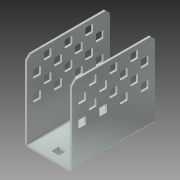
# Autodesk Inventor part: 276-1926
Saved by Autodesk Inventor 2013 (Build 170138000, 138)
## iProperties
Category: Motion
Company: Autodesk Inc.
Created: 2012-02-28
Part Number: 276-1926
Material: Steel
Document SubType Name: Sheet Metal
Designer: Autodesk Inc.
Density: 7.85 g/cm^3
Sheet Metal Rule: Default
Catalog Web Link: http://www.vexrobotics.com/276-1926.html
Vendor: VEX
Author: Autodesk Inc.
Autodesk Inventor part; units mm, degrees
ref_plane "YZ Plane" through (0, 0, 0) normal (1, 0, 0) x (0, 1, 0)
ref_plane "XZ Plane" through (0, 0, 0) normal (0, 1, 0) x (-1, 0, 0)
ref_plane "XY Plane" through (0, 0, 0) normal (0, 0, 1) x (1, 0, 0)
sketch "Sketch1" plane through (0, 0, 0) normal (0, 0, 1) x (1, 0, 0)
  line L0 (0, 0) -> (50.8, 0)
  line L1 (50.8, 0) -> (50.8, 28.6766)
  line L2 (50.8, 28.6766) -> (0, 28.6766)
  line L3 (0, 28.6766) -> (0, 0)
  dimension "d0" = 50.8
  dimension "d1" = 28.6766
  measures "d0" distance of L2.end L1.end
  measures "d1" distance of L1.end L0.end
extrude "Plate1" add sketch "Sketch1" against normal blind 1.19
sketch "Sketch2" plane through (50.8, 1.19, -1.19) normal (0, -1, 0) x (1, 0, 0)
  line L0 (-50.8, 0) -> (0, 0)
  line L1 (0, 0) -> (0, 47.879)
  line L2 (0, 47.879) -> (-50.8, 47.879)
  line L3 (-50.8, 47.879) -> (-50.8, 0)
  constraints: 6 end point, 1 horizontal, 1 perpendicular, 1 vertical
edge flange "Flange1" height 47.879 angle 90 thickness 1.19 bend radius 1.19 thickness toward (0, -1, 0) relief straight relief width 1.19 relief depth 0.595 corner gap 1.19 corner form 0 edges at (25.4, 0, 0) (25.4, 28.6766, 0) wall of the first edge with corners at (0, 1.19, -1.19) (50.8, 1.19, -1.19) (50.8, 1.19, 46.689) (0, 1.19, 46.689)
bend "Bend1"
corner "Corner1"
chamfer "Corner Chamfer1" distance 2.54 angle 45 4 edges at (0, 28.0816, 46.689) (0, 0.595, 46.689) (50.8, 28.0816, 46.689) (50.8, 0.595, 46.689)
sketch "Sketch3" plane through (0, 0, 1.19) normal (0, -1, 0) x (1, 0, 0)
  line L0 (2.54, 45.499) -> (48.26, 45.499) projected
  line L1 (0, 0) -> (0, 42.959) projected
  line L2 (10.8966, 37.9552) -> (14.5034, 37.9552)
  line L3 (15.0114, 38.4632) -> (15.0114, 42.07)
  line L4 (14.5034, 42.578) -> (10.8966, 42.578)
  line L5 (10.3886, 42.07) -> (10.3886, 38.4632)
  line L6 (12.7, 37.9552) -> (12.7, 42.578) construction
  line L7 (10.3886, 40.2666) -> (15.0114, 40.2666) construction
  arc A0 (10.8966, 42.578) -> (10.3886, 42.07) centre (10.8966, 42.07) ccw
  arc A1 (15.0114, 42.07) -> (14.5034, 42.578) centre (14.5034, 42.07) ccw
  arc A2 (14.5034, 37.9552) -> (15.0114, 38.4632) centre (14.5034, 38.4632) ccw
  arc A3 (10.3886, 38.4632) -> (10.8966, 37.9552) centre (10.8966, 38.4632) ccw
  line L8 (23.5966, 37.9552) -> (27.2034, 37.9552)
  line L9 (27.7114, 38.4632) -> (27.7114, 42.07)
  line L10 (27.2034, 42.578) -> (23.5966, 42.578)
  line L11 (23.0886, 42.07) -> (23.0886, 38.4632)
  line L12 (25.4, 37.9552) -> (25.4, 42.578) construction
  line L13 (23.0886, 40.2666) -> (27.7114, 40.2666) construction
  arc A4 (23.5966, 42.578) -> (23.0886, 42.07) centre (23.5966, 42.07) ccw
  arc A5 (27.7114, 42.07) -> (27.2034, 42.578) centre (27.2034, 42.07) ccw
  arc A6 (27.2034, 37.9552) -> (27.7114, 38.4632) centre (27.2034, 38.4632) ccw
  arc A7 (23.0886, 38.4632) -> (23.5966, 37.9552) centre (23.5966, 38.4632) ccw
  line L14 (36.2966, 37.9552) -> (39.9034, 37.9552)
  line L15 (40.4114, 38.4632) -> (40.4114, 42.07)
  line L16 (39.9034, 42.578) -> (36.2966, 42.578)
  line L17 (35.7886, 42.07) -> (35.7886, 38.4632)
  line L18 (38.1, 37.9552) -> (38.1, 42.578) construction
  line L19 (35.7886, 40.2666) -> (40.4114, 40.2666) construction
  arc A8 (36.2966, 42.578) -> (35.7886, 42.07) centre (36.2966, 42.07) ccw
  arc A9 (40.4114, 42.07) -> (39.9034, 42.578) centre (39.9034, 42.07) ccw
  arc A10 (39.9034, 37.9552) -> (40.4114, 38.4632) centre (39.9034, 38.4632) ccw
  arc A11 (35.7886, 38.4632) -> (36.2966, 37.9552) centre (36.2966, 38.4632) ccw
  line L20 (10.8966, 25.2552) -> (14.5034, 25.2552)
  line L21 (15.0114, 25.7632) -> (15.0114, 29.37)
  line L22 (14.5034, 29.878) -> (10.8966, 29.878)
  line L23 (10.3886, 29.37) -> (10.3886, 25.7632)
  line L24 (12.7, 25.2552) -> (12.7, 29.878) construction
  line L25 (10.3886, 27.5666) -> (15.0114, 27.5666) construction
  arc A12 (10.8966, 29.878) -> (10.3886, 29.37) centre (10.8966, 29.37) ccw
  arc A13 (15.0114, 29.37) -> (14.5034, 29.878) centre (14.5034, 29.37) ccw
  arc A14 (14.5034, 25.2552) -> (15.0114, 25.7632) centre (14.5034, 25.7632) ccw
  arc A15 (10.3886, 25.7632) -> (10.8966, 25.2552) centre (10.8966, 25.7632) ccw
  line L26 (23.5966, 25.2552) -> (27.2034, 25.2552)
  line L27 (27.7114, 25.7632) -> (27.7114, 29.37)
  arc A16 (23.0886, 25.7632) -> (23.5966, 25.2552) centre (23.5966, 25.7632) ccw
  arc A17 (27.7114, 29.37) -> (27.2034, 29.878) centre (27.2034, 29.37) ccw
  line L28 (23.0886, 27.5666) -> (27.7114, 27.5666) construction
  line L29 (25.4, 25.2552) -> (25.4, 29.878) construction
  line L30 (23.0886, 29.37) -> (23.0886, 25.7632)
  arc A18 (23.5966, 29.878) -> (23.0886, 29.37) centre (23.5966, 29.37) ccw
  arc A19 (27.2034, 25.2552) -> (27.7114, 25.7632) centre (27.2034, 25.7632) ccw
  line L31 (27.2034, 29.878) -> (23.5966, 29.878)
  line L32 (36.2966, 25.2552) -> (39.9034, 25.2552)
  line L33 (40.4114, 25.7632) -> (40.4114, 29.37)
  arc A20 (35.7886, 25.7632) -> (36.2966, 25.2552) centre (36.2966, 25.7632) ccw
  arc A21 (40.4114, 29.37) -> (39.9034, 29.878) centre (39.9034, 29.37) ccw
  line L34 (35.7886, 27.5666) -> (40.4114, 27.5666) construction
  line L35 (38.1, 25.2552) -> (38.1, 29.878) construction
  line L36 (35.7886, 29.37) -> (35.7886, 25.7632)
  arc A22 (36.2966, 29.878) -> (35.7886, 29.37) centre (36.2966, 29.37) ccw
  arc A23 (39.9034, 25.2552) -> (40.4114, 25.7632) centre (39.9034, 25.7632) ccw
  line L37 (39.9034, 29.878) -> (36.2966, 29.878)
  line L38 (4.5466, 31.6052) -> (8.1534, 31.6052)
  line L39 (8.6614, 32.1132) -> (8.6614, 35.72)
  line L40 (8.1534, 36.228) -> (4.5466, 36.228)
  line L41 (4.0386, 35.72) -> (4.0386, 32.1132)
  arc A24 (4.0386, 32.1132) -> (4.5466, 31.6052) centre (4.5466, 32.1132) ccw
  arc A25 (4.5466, 36.228) -> (4.0386, 35.72) centre (4.5466, 35.72) ccw
  arc A26 (8.6614, 35.72) -> (8.1534, 36.228) centre (8.1534, 35.72) ccw
  arc A27 (8.1534, 31.6052) -> (8.6614, 32.1132) centre (8.1534, 32.1132) ccw
  line L42 (6.35, 31.6052) -> (6.35, 36.228) construction
  line L43 (4.0386, 33.9166) -> (8.6614, 33.9166) construction
  line L44 (17.2466, 31.6052) -> (20.8534, 31.6052)
  line L45 (21.3614, 32.1132) -> (21.3614, 35.72)
  line L46 (20.8534, 36.228) -> (17.2466, 36.228)
  line L47 (16.7386, 35.72) -> (16.7386, 32.1132)
  arc A28 (16.7386, 32.1132) -> (17.2466, 31.6052) centre (17.2466, 32.1132) ccw
  arc A29 (17.2466, 36.228) -> (16.7386, 35.72) centre (17.2466, 35.72) ccw
  arc A30 (21.3614, 35.72) -> (20.8534, 36.228) centre (20.8534, 35.72) ccw
  arc A31 (20.8534, 31.6052) -> (21.3614, 32.1132) centre (20.8534, 32.1132) ccw
  line L48 (19.05, 31.6052) -> (19.05, 36.228) construction
  line L49 (16.7386, 33.9166) -> (21.3614, 33.9166) construction
  line L50 (29.9466, 31.6052) -> (33.5534, 31.6052)
  line L51 (34.0614, 32.1132) -> (34.0614, 35.72)
  line L52 (33.5534, 36.228) -> (29.9466, 36.228)
  line L53 (29.4386, 35.72) -> (29.4386, 32.1132)
  arc A32 (29.4386, 32.1132) -> (29.9466, 31.6052) centre (29.9466, 32.1132) ccw
  arc A33 (29.9466, 36.228) -> (29.4386, 35.72) centre (29.9466, 35.72) ccw
  arc A34 (34.0614, 35.72) -> (33.5534, 36.228) centre (33.5534, 35.72) ccw
  arc A35 (33.5534, 31.6052) -> (34.0614, 32.1132) centre (33.5534, 32.1132) ccw
  line L54 (31.75, 31.6052) -> (31.75, 36.228) construction
  line L55 (29.4386, 33.9166) -> (34.0614, 33.9166) construction
  line L56 (42.6466, 31.6052) -> (46.2534, 31.6052)
  line L57 (46.7614, 32.1132) -> (46.7614, 35.72)
  line L58 (46.2534, 36.228) -> (42.6466, 36.228)
  line L59 (42.1386, 35.72) -> (42.1386, 32.1132)
  arc A36 (42.1386, 32.1132) -> (42.6466, 31.6052) centre (42.6466, 32.1132) ccw
  arc A37 (42.6466, 36.228) -> (42.1386, 35.72) centre (42.6466, 35.72) ccw
  arc A38 (46.7614, 35.72) -> (46.2534, 36.228) centre (46.2534, 35.72) ccw
  arc A39 (46.2534, 31.6052) -> (46.7614, 32.1132) centre (46.2534, 32.1132) ccw
  line L60 (44.45, 31.6052) -> (44.45, 36.228) construction
  line L61 (42.1386, 33.9166) -> (46.7614, 33.9166) construction
  line L62 (4.5466, 18.9052) -> (8.1534, 18.9052)
  line L63 (8.6614, 19.4132) -> (8.6614, 23.02)
  line L64 (8.1534, 23.528) -> (4.5466, 23.528)
  line L65 (4.0386, 23.02) -> (4.0386, 19.4132)
  arc A40 (4.0386, 19.4132) -> (4.5466, 18.9052) centre (4.5466, 19.4132) ccw
  arc A41 (4.5466, 23.528) -> (4.0386, 23.02) centre (4.5466, 23.02) ccw
  arc A42 (8.6614, 23.02) -> (8.1534, 23.528) centre (8.1534, 23.02) ccw
  arc A43 (8.1534, 18.9052) -> (8.6614, 19.4132) centre (8.1534, 19.4132) ccw
  line L66 (6.35, 18.9052) -> (6.35, 23.528) construction
  line L67 (4.0386, 21.2166) -> (8.6614, 21.2166) construction
  line L68 (17.2466, 18.9052) -> (20.8534, 18.9052)
  line L69 (21.3614, 19.4132) -> (21.3614, 23.02)
  line L70 (20.8534, 23.528) -> (17.2466, 23.528)
  line L71 (16.7386, 23.02) -> (16.7386, 19.4132)
  arc A44 (16.7386, 19.4132) -> (17.2466, 18.9052) centre (17.2466, 19.4132) ccw
  arc A45 (17.2466, 23.528) -> (16.7386, 23.02) centre (17.2466, 23.02) ccw
  arc A46 (21.3614, 23.02) -> (20.8534, 23.528) centre (20.8534, 23.02) ccw
  arc A47 (20.8534, 18.9052) -> (21.3614, 19.4132) centre (20.8534, 19.4132) ccw
  line L72 (19.05, 18.9052) -> (19.05, 23.528) construction
  line L73 (16.7386, 21.2166) -> (21.3614, 21.2166) construction
  line L74 (29.9466, 18.9052) -> (33.5534, 18.9052)
  line L75 (34.0614, 19.4132) -> (34.0614, 23.02)
  line L76 (33.5534, 23.528) -> (29.9466, 23.528)
  line L77 (29.4386, 23.02) -> (29.4386, 19.4132)
  arc A48 (29.4386, 19.4132) -> (29.9466, 18.9052) centre (29.9466, 19.4132) ccw
  arc A49 (29.9466, 23.528) -> (29.4386, 23.02) centre (29.9466, 23.02) ccw
  arc A50 (34.0614, 23.02) -> (33.5534, 23.528) centre (33.5534, 23.02) ccw
  arc A51 (33.5534, 18.9052) -> (34.0614, 19.4132) centre (33.5534, 19.4132) ccw
  line L78 (31.75, 18.9052) -> (31.75, 23.528) construction
  line L79 (29.4386, 21.2166) -> (34.0614, 21.2166) construction
  line L80 (42.6466, 18.9052) -> (46.2534, 18.9052)
  line L81 (46.7614, 19.4132) -> (46.7614, 23.02)
  line L82 (46.2534, 23.528) -> (42.6466, 23.528)
  line L83 (42.1386, 23.02) -> (42.1386, 19.4132)
  arc A52 (42.1386, 19.4132) -> (42.6466, 18.9052) centre (42.6466, 19.4132) ccw
  arc A53 (42.6466, 23.528) -> (42.1386, 23.02) centre (42.6466, 23.02) ccw
  arc A54 (46.7614, 23.02) -> (46.2534, 23.528) centre (46.2534, 23.02) ccw
  arc A55 (46.2534, 18.9052) -> (46.7614, 19.4132) centre (46.2534, 19.4132) ccw
  line L84 (44.45, 18.9052) -> (44.45, 23.528) construction
  line L85 (42.1386, 21.2166) -> (46.7614, 21.2166) construction
  point P0 (0, -1.19)
  point P1 (15.0114, 42.578)
  point P2 (15.0114, 37.9552)
  point P3 (10.3886, 42.578)
  point P4 (27.7114, 42.578)
  point P5 (27.7114, 37.9552)
  point P6 (23.0886, 42.578)
  point P7 (40.4114, 42.578)
  point P8 (40.4114, 37.9552)
  point P9 (35.7886, 42.578)
  point P10 (15.0114, 29.878)
  point P11 (15.0114, 25.2552)
  point P12 (10.3886, 29.878)
  point P13 (27.7114, 25.2552)
  point P14 (27.7114, 29.878)
  point P15 (23.0886, 29.878)
  point P16 (40.4114, 25.2552)
  point P17 (40.4114, 29.878)
  point P18 (35.7886, 29.878)
  dimension "d16" = 4.6228
  dimension "d17" = 4.6228
  dimension "d18" = 0.508
  dimension "d19" = 12.7
  dimension "d20" = 5.2324
  dimension "d23" = 12.7
  dimension "d30" = 12.7
  dimension "d35" = 0.508
  dimension "d36" = 6.35
  dimension "d37" = 4.6228
  dimension "d38" = 4.6228
  dimension "d39" = 6.35
  dimension "d42" = 12.7
  dimension "d45" = 12.7
  constraints: 168 end point, 112 point on circle, 56 centre point, 36 point on line, 16 tangent, 8 midpoint, 6 equal radius, 4 horizontal, 4 parallel, 2 perpendicular, 2 vertical, 327 other
  measures "d16" distance of point (10.389, 42.578) point (15.011, 42.578)
  measures "d17" distance of point (15.011, 42.578) point (15.011, 37.955)
  measures "d18" radius of A0
  measures "d19" distance between parallel lines of L6 L1
  measures "d20" distance between parallel lines of L7 L0
  measures "d23" distance of point (15.011, 37.955) point (27.711, 37.955)
  measures "d30" distance of L4.start L22.start
  measures "d35" radius of A24
  measures "d36" distance between parallel lines of L42 L1
  measures "d37" distance between parallel lines of L38 L40
  measures "d38" distance between parallel lines of L39 L41
  measures "d39" distance between parallel lines of L43 L7
  measures "d42" distance of L39.end L45.end
  measures "d45" distance of L39.end L63.end
extrude "Cut1" cut sketch "Sketch3" against normal blind 1.19
ref_plane "Work Plane1" through (0, 14.3383, 1.19) normal (0, -1, 0) x (1, 0, 0)
mirror "Mirror1" about plane through (0, 14.3383, 1.19) normal (0, -1, 0) of "Cut1"
sketch "Sketch4" plane through (0, 0, -1.19) normal (0, 0, -1) x (-1, 0, 0)
  line L0 (-50.8, 2.38) -> (0, 2.38) projected
  line L1 (0, 26.2966) -> (0, 2.38) projected
  line L2 (-4.5466, 16.6497) -> (-8.1534, 16.6497)
  line L3 (-8.6614, 16.1417) -> (-8.6614, 12.5349)
  line L4 (-8.1534, 12.0269) -> (-4.5466, 12.0269)
  line L5 (-4.0386, 12.5349) -> (-4.0386, 16.1417)
  arc A0 (-4.5466, 12.0269) -> (-4.0386, 12.5349) centre (-4.5466, 12.5349) ccw
  arc A1 (-8.6614, 12.5349) -> (-8.1534, 12.0269) centre (-8.1534, 12.5349) ccw
  arc A2 (-8.1534, 16.6497) -> (-8.6614, 16.1417) centre (-8.1534, 16.1417) ccw
  arc A3 (-4.0386, 16.1417) -> (-4.5466, 16.6497) centre (-4.5466, 16.1417) ccw
  line L6 (-6.35, 16.6497) -> (-6.35, 12.0269) construction
  line L7 (-17.2466, 16.6497) -> (-20.8534, 16.6497)
  line L8 (-21.3614, 16.1417) -> (-21.3614, 12.5349)
  line L9 (-20.8534, 12.0269) -> (-17.2466, 12.0269)
  line L10 (-16.7386, 12.5349) -> (-16.7386, 16.1417)
  arc A4 (-17.2466, 12.0269) -> (-16.7386, 12.5349) centre (-17.2466, 12.5349) ccw
  arc A5 (-21.3614, 12.5349) -> (-20.8534, 12.0269) centre (-20.8534, 12.5349) ccw
  arc A6 (-20.8534, 16.6497) -> (-21.3614, 16.1417) centre (-20.8534, 16.1417) ccw
  arc A7 (-16.7386, 16.1417) -> (-17.2466, 16.6497) centre (-17.2466, 16.1417) ccw
  line L11 (-19.05, 16.6497) -> (-19.05, 12.0269) construction
  line L12 (-29.9466, 16.6497) -> (-33.5534, 16.6497)
  line L13 (-34.0614, 16.1417) -> (-34.0614, 12.5349)
  line L14 (-33.5534, 12.0269) -> (-29.9466, 12.0269)
  line L15 (-29.4386, 12.5349) -> (-29.4386, 16.1417)
  arc A8 (-29.9466, 12.0269) -> (-29.4386, 12.5349) centre (-29.9466, 12.5349) ccw
  arc A9 (-34.0614, 12.5349) -> (-33.5534, 12.0269) centre (-33.5534, 12.5349) ccw
  arc A10 (-33.5534, 16.6497) -> (-34.0614, 16.1417) centre (-33.5534, 16.1417) ccw
  arc A11 (-29.4386, 16.1417) -> (-29.9466, 16.6497) centre (-29.9466, 16.1417) ccw
  line L16 (-31.75, 16.6497) -> (-31.75, 12.0269) construction
  line L17 (-42.6466, 16.6497) -> (-46.2534, 16.6497)
  line L18 (-46.7614, 16.1417) -> (-46.7614, 12.5349)
  line L19 (-46.2534, 12.0269) -> (-42.6466, 12.0269)
  line L20 (-42.1386, 12.5349) -> (-42.1386, 16.1417)
  arc A12 (-42.6466, 12.0269) -> (-42.1386, 12.5349) centre (-42.6466, 12.5349) ccw
  arc A13 (-46.7614, 12.5349) -> (-46.2534, 12.0269) centre (-46.2534, 12.5349) ccw
  arc A14 (-46.2534, 16.6497) -> (-46.7614, 16.1417) centre (-46.2534, 16.1417) ccw
  arc A15 (-42.1386, 16.1417) -> (-42.6466, 16.6497) centre (-42.6466, 16.1417) ccw
  line L21 (-44.45, 16.6497) -> (-44.45, 12.0269) construction
  point P0 (0, 0)
  point P1 (-4.0386, 14.3383)
  point P2 (0, 14.3383)
  point P3 (-16.7386, 14.3383)
  point P4 (-29.4386, 14.3383)
  point P5 (-42.1386, 14.3383)
  dimension "d50" = 4.6228
  dimension "d51" = 4.6228
  dimension "d52" = 0.508
  dimension "d53" = 6.35
  dimension "d56" = 12.7
  constraints: 40 end point, 32 point on circle, 16 centre point, 8 tangent, 4 midpoint, 3 equal radius, 2 horizontal, 2 parallel, 1 horizontal alignment, 1 perpendicular, 72 other
  measures "d50" distance between parallel lines of L2 L4
  measures "d51" distance between parallel lines of L5 L3
  measures "d52" radius of A0
  measures "d53" distance between parallel lines of L6 L1
  measures "d56" distance of L5.end L10.end
extrude "Cut2" cut sketch "Sketch4" against normal blind 1.19
sketch "Sketch5" plane through (0, 0, 1.19) normal (0, -1, 0) x (1, 0, 0)
  line L0 (10.8966, 42.578) -> (14.5034, 42.578) projected
  line L1 (15.0114, 42.07) -> (15.0114, 38.4632) projected
  line L2 (14.5034, 37.9552) -> (10.8966, 37.9552) projected
  line L3 (10.3886, 38.4632) -> (10.3886, 42.07) projected
  circle A0 centre (12.7, 40.2666) radius 2.3114
  point P0 (0, -1.19)
  constraints: 4 tangent, 1 centre point
surface extrude "ExtrusionSrf1" sketch "Sketch5" against normal up to surface (1.19 mm away) shown no curves A0
pattern_linear "Rectangular Pattern1" count 3 spacing 12.7 along (1, 0, 0) count 2 spacing 12.7 along (0, 0, -1) of "ExtrusionSrf1"
sketch "Sketch6" plane through (0, 0, 1.19) normal (0, -1, 0) x (1, 0, 0)
  line L0 (8.1534, 31.6052) -> (4.5466, 31.6052) projected
  line L1 (4.0386, 32.1132) -> (4.0386, 35.72) projected
  line L2 (4.5466, 36.228) -> (8.1534, 36.228) projected
  line L3 (8.6614, 35.72) -> (8.6614, 32.1132) projected
  circle A0 centre (6.35, 33.9166) radius 2.3114
  point P0 (0, -1.19)
  constraints: 4 tangent, 1 centre point
surface extrude "ExtrusionSrf7" sketch "Sketch6" against normal up to surface (1.19 mm away) shown no curves A0
pattern_linear "Rectangular Pattern2" count 4 spacing 12.7 along (1, 0, 0) count 2 spacing 12.7 along (0, 0, -1) of "ExtrusionSrf7"
ref_plane "Work Plane2" through (0, 14.3383, 0) normal (0, -1, 0) x (1, 0, 0)
mirror "Mirror2" about plane through (0, 14.3383, 0) normal (0, -1, 0) of "ExtrusionSrf7", "Rectangular Pattern2", "ExtrusionSrf1", "Rectangular Pattern1"
sketch "Sketch7" plane through (0, 0, 0) normal (0, 0, 1) x (1, 0, 0)
  line L0 (4.0386, 12.5349) -> (4.0386, 16.1417) projected
  line L1 (4.5466, 16.6497) -> (8.1534, 16.6497) projected
  line L2 (8.6614, 16.1417) -> (8.6614, 12.5349) projected
  line L3 (8.1534, 12.0269) -> (4.5466, 12.0269) projected
  circle A0 centre (6.35, 14.3383) radius 2.3114
  point P0 (0, 0)
  constraints: 4 tangent, 1 centre point
surface extrude "ExtrusionSrf29" sketch "Sketch7" against normal up to surface (1.19 mm away) shown no curves A0
pattern_linear "Rectangular Pattern3" count 4 spacing 12.7 along (1, 0, 0) of "ExtrusionSrf29"
equation "\"d48\" = Thickness"
equation "\"d51\" = d50"
equation "\"d61\" = Thickness"
equation "\"d3\" = BendReliefWidth"
equation "\"d4\" = BendReliefDepth"
equation "\"d5\" = MinimumRemnant"
equation "\"d6\" = BendRadius"
equation "\"d9\" = BendRadius"
equation "\"d10\" = CornerReliefSize"
equation "\"d11\" = GapSize"
equation "\"d12\" = JacobiRadiusSize"
equation "\"BendRadius\" = Thickness"
equation "\"BendReliefWidth\" = Thickness"
equation "\"BendReliefDepth\" = 0.5 * Thickness"
equation "\"CornerReliefSize\" = 4 * Thickness"
equation "\"MinimumRemnant\" = 2 * Thickness"
equation "\"TransitionRadius\" = BendRadius"
equation "\"JacobiRadiusSize\" = BendRadius"
equation "\"GapSize\" = Thickness"
equation "\"d2\" = BendRadius"
equation "\"Thickness\" = 1.19"
body "Solid1"
body "Srf1"
body "Srf2"
body "Srf3"
body "Srf4"
body "Srf5"
body "Srf6"
body "Srf7"
body "Srf8"
body "Srf9"
body "Srf10"
body "Srf11"
body "Srf12"
body "Srf13"
body "Srf14"
body "Srf18"
body "Srf19"
body "Srf20"
body "Srf15"
body "Srf16"
body "Srf17"
body "Srf21"
body "Srf22"
body "Srf23"
body "Srf24"
body "Srf25"
body "Srf26"
body "Srf27"
body "Srf28"
body "Srf29"
body "Srf30"
body "Srf31"
body "Srf32"
